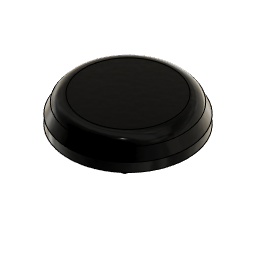
Suitcase v18 (Autodesk Fusion 360 archive; units mm, degrees)
design "LTE Antenna 202-4091"
Autodesk Fusion 360 part; units mm, degrees
(part 1 of 2)
sketch "Sketch1" plane through (0, 0, 0) normal (0, 1, 0) x (1, 0, 0)
  line L0 (0, 0) -> (0, -60.7821)
  line L1 (0, -15.2) -> (30, -15.2)
  line L2 (30, -15.2) -> (34.5, -5)
  line L3 (34.5, -5) -> (34.5, 0)
  line L4 (0, 0) -> (0, 30)
  line L5 (34.5, 0) -> (7.25, 0)
  line L6 (7.25, 0) -> (7.25, 19.3)
  line L7 (7.25, 19.3) -> (0, 19.3)
  dimension "d1" = 69
  dimension "d2" = 15.2
  dimension "d4" = 60
  dimension "d5" = 5
  dimension "d6" = 14.5
  dimension "d7" = 19.3
  constraint coincident L0.start L4.start
  constraint vertical L0
  constraint coincident L0 L1.start
  constraint perpendicular L0 L1
  constraint perpendicular L1 L3
  constraint parallel L0 L4
  constraint perpendicular L3 L5
  constraint perpendicular L5 L6
  constraint coincident L4 L7.end
  constraint perpendicular L4 L7
  constraint coincident L0.start L5
  measures "d2" distance of L0.start L1
  measures "d5" distance of L2.end L3.end
  measures "d7" distance of L5 L7
revolve "Revolve1" add sketch "Sketch1" angle 360 about axis through (0, 0, 0) along (0, 0, 1) makes body 1
fillet "Fillet1" radius 7 1 edges at (-27.9698, -10.8485, 15.2) on bodies 1
sketch "Sketch2" plane through (0, 0, -19.3) normal (0, 0, -1) x (1, 0, 0)
  circle A0 centre (0, 0) radius 7.25
  line L0 (2.75, 0) -> (2.75, 7.25)
  arc A1 (2.75, 7.25) -> (-2.75, 7.25) centre (0, 7.25) ccw
  line L1 (-2.75, 7.25) -> (-2.75, 0)
  arc A2 (-2.75, 0) -> (2.75, 0) centre (0, 0) ccw
  line L2 (0, 0) -> (0, 7.25) construction
  dimension "d11" = 5.5
  constraint tangent L0 A1
  constraint tangent A1 L1
  constraint parallel L0 L1
  constraint tangent L1 A2
  constraint tangent L0 A2
  constraint coincident A0 A1.centre
  constraint vertical L2
  constraint coincident A0.centre A2.centre
  measures "d11" distance of L0 L1
sketch "Sketch3" plane through (0, 0, 0) normal (0, 0, -1) x (1, 0, 0)
  circle A0 centre (0, 0) radius 7.25
  circle A1 centre (0, 0) radius 34.5
  line L0 (-7.25, 7.25) -> (7.25, 7.25)
  line L1 (7.25, 7.25) -> (7.25, -7.25)
  line L2 (7.25, -7.25) -> (-7.25, -7.25)
  line L3 (-7.25, -7.25) -> (-7.25, 7.25)
  circle A2 centre (0, 0) radius 7.25
  constraint horizontal L0
  constraint vertical L1
  constraint horizontal L2
  constraint vertical L3
  constraint tangent L1 A2
  constraint tangent L2 A2
  constraint tangent L3 A2
  constraint tangent L0 A2
extrude "Extrude1" add sketch "Sketch3" along normal blind 2.7 separate body contours A0 A2 | A0 L1 L2 A2 | A0 L0 L1 A2 | A0 L0 L3 A2 | A0 L2 L3 A2 makes body 2
extrude "Extrude2" cut sketch "Sketch2" against normal up to surface (19.3 mm away) contours A0 L0 L1 A2 | A0 L0 A1 L1 picked at (0, 2.4167) bodies 2 1
sketch "Sketch1 (2)" plane through (0, 0, 0) normal (0, 0, 1) x (1, 0, 0) in component "NUT"
  line L0 (11, -6.3509) -> (11, 6.3509)
  line L1 (11, 6.3509) -> (0, 12.7017)
  line L2 (0, 12.7017) -> (-11, 6.3509)
  line L3 (-11, 6.3509) -> (-11, -6.3509)
  line L4 (-11, -6.3509) -> (0, -12.7017)
  line L5 (0, -12.7017) -> (11, -6.3509)
  circle A0 centre (0, 0) radius 7.25
  dimension "d16" = 11
  dimension "d17" = 14.5
  constraint coincident A0.centre origin
  constraint vertical L0
  measures "d16" distance of A0.centre L5
  measures "d17" diameter of A0
extrude "Extrude1'" add sketch "Sketch1 (2)" against normal blind 5.6 separate body makes body 3 in component "NUT"
sketch "Sketch2 (2)" plane through (0, 0, 0) normal (0, 1, 0) x (1, 0, 0) in component "NUT"
  line L0 (0, 0) -> (10.6333, 0)
  line L1 (10.6333, 0) -> (13, 0)
  line L2 (13, 0) -> (13, -6.6)
  line L3 (13, -6.6) -> (12.2, -6.6)
  line L4 (12.2, -6.6) -> (12.2, -0.8)
  line L5 (12.2, -0.8) -> (7.5, -0.8)
  line L6 (7.5, -0.8) -> (7.5, 0)
  line L7 (0, 0) -> (0, -13)
  dimension "d20" = 6.6
  dimension "d21" = 15
  dimension "d22" = 26
  dimension "d23" = 0.8
  dimension "d24" = 0.8
  constraint coincident L0.start L7.start
  constraint horizontal L0
  constraint parallel L0 L1
  constraint perpendicular L1 L2
  constraint perpendicular L2 L3
  constraint perpendicular L3 L4
  constraint perpendicular L4 L5
  constraint coincident L0 L6.end
  constraint perpendicular L0 L6
  constraint perpendicular L0 L7
  measures "d20" distance of L1.end L2.end
  measures "d23" distance of L2 L4
  measures "d24" distance of L1 L5
revolve "Revolve1'" add sketch "Sketch2 (2)" angle 360 about axis through (0, 0, 0) along (0, 0, 1) bodies 3 in component "NUT"
sketch "Sketch3 (2)" plane through (0, 0, 0) normal (0, 1, 0) x (1, 0, 0) in component "NUT"
  line L0 (0, 0) -> (0, -11.559) construction
  line L1 (-9.7763, -5) -> (-1.7, -5)
  line L2 (-1.7, -5) -> (0, -6.7)
  line L3 (0, -6.7) -> (1.7, -5)
  line L4 (1.7, -5) -> (9.7763, -5)
  line L5 (9.7763, -5) -> (9.7763, -9.682)
  line L6 (9.7763, -9.682) -> (-9.7763, -9.682)
  line L7 (-9.7763, -9.682) -> (-9.7763, -5)
  dimension "d26" = 45
  dimension "d28" = 5
  dimension "d29" = 6.7
  dimension "d30" = 19.5526
  dimension "d31" = 4.682
  constraint coincident L0.start origin
  constraint vertical L0
  constraint horizontal L1
  constraint coincident L0 L2.end
  constraint perpendicular L0 L4
  constraint perpendicular L4 L5
  constraint perpendicular L5 L6
  constraint symmetric L0 L2 L3
  constraint collinear L1 L4
  constraint symmetric L0 L5 L7
  measures "d26" angle of L0 L2
  measures "d28" distance of L0.start L4
  measures "d29" distance of L0.start L2.end
  measures "d30" distance of L5 L7
  measures "d31" distance of L4 L6
extrude "Extrude2'" cut sketch "Sketch3 (2)" against normal blind 22 bodies 3 in component "NUT"
pattern_circular "C-Pattern1" count 4 over 360 about axis through (0, 0, 1.75) along (0, 0, 1) of "Extrude2'" in component "NUT"
component "NUT" placed x (1, 0, 0) y (0, 1, 0) z (0, 0, 1) at (0, 0, -10.4)
equation "d16 = 22 mm / 2"

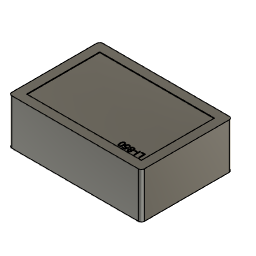
design "LICOR_850A"
Autodesk Fusion 360 part; units mm, degrees
sketch "Sketch1" plane through (0, 0, 0) normal (0, 0, 1) x (1, 0, 0)
  line L0 (0, 0) -> (222.3, 0)
  line L1 (222.3, 0) -> (222.3, 152.5)
  line L2 (222.3, 152.5) -> (0, 152.5)
  line L3 (0, 152.5) -> (0, 0)
  dimension "d1" = 222.3
  dimension "d2" = 152.5
  constraint horizontal L0
  constraint vertical L1
  constraint horizontal L2
  constraint vertical L3
  constraint coincident L0.start L3.end
  measures "d1" distance of L0.start L0.end
  measures "d2" distance of L0.start L2.end
extrude "Extrude1" add sketch "Sketch1" along normal blind 76.2
sketch "Sketch2" plane through (0, 0, 76.2) normal (0, 0, 1) x (-1, 0, 0)
  line L0 (0, -152.5) -> (0, 0)
  line L1 (0, 0) -> (-222.3, 0)
  line L2 (-222.3, 0) -> (-222.3, -152.5)
  line L3 (-222.3, -152.5) -> (0, -152.5)
fillet "Fillet1" radius 5 4 edges at (222.3, 0, 38.1) (0, 152.5, 38.1) (222.3, 152.5, 38.1) (0, 0, 38.1)
sketch "Sketch3" plane through (0, 0, 76.2) normal (0, 0, 1) x (-1, 0, 0)
  arc A0 (0, -5) -> (-5, 0) centre (-5, -5) ccw
  line L0 (-5, 0) -> (-217.3, 0)
  arc A1 (-217.3, 0) -> (-222.3, -5) centre (-217.3, -5) ccw
  line L1 (-222.3, -5) -> (-222.3, -147.5)
  arc A2 (-222.3, -147.5) -> (-217.3, -152.5) centre (-217.3, -147.5) ccw
  line L2 (-217.3, -152.5) -> (-5, -152.5)
  arc A3 (-5, -152.5) -> (0, -147.5) centre (-5, -147.5) ccw
  line L3 (0, -147.5) -> (0, -5)
  line L4 (-207.3, -15) -> (-207.3, -137.5)
  line L5 (-207.3, -137.5) -> (-15, -137.5)
  line L6 (-15, -137.5) -> (-15, -15)
  line L7 (-15, -15) -> (-207.3, -15)
  dimension "d7" = -15
extrude "Extrude2" cut sketch "Sketch3" against normal blind 1 contours L4 L5 L6 L7
sketch "Sketch4" plane through (0, 152.5, 0) normal (0, 1, 0) x (-1, 0, 0)
  line L0 (-217.3, 76.2) -> (-217.3, 0)
  line L1 (-217.3, 0) -> (-5, 0)
  line L2 (-5, 0) -> (-5, 76.2)
  line L3 (-5, 76.2) -> (-217.3, 76.2)
  line L4 (-135.3, 0) -> (-135.3, 76.2) construction
  circle A0 centre (-135.3, 30) radius 6
  line L5 (-111.15, 76.2) -> (-111.15, 0) construction
  circle A1 centre (-96, 30) radius 6
  line L6 (-201.4, 35) -> (-182.4, 35)
  line L7 (-182.4, 35) -> (-182.4, 25.3) construction
  line L8 (-182.4, 25.3) -> (-201.4, 25.3)
  line L9 (-201.4, 25.3) -> (-201.4, 35) construction
  line L10 (-201.4, 35) -> (-199.4, 25.3)
  line L11 (-182.4, 35) -> (-184.4, 25.3)
  circle A2 centre (-176.9, 30.15) radius 2.5
  line L12 (-191.9, 35) -> (-191.9, 25.3) construction
  line L13 (-191.9, 30.15) -> (-176.9, 30.15) construction
  circle A3 centre (-206.9, 30.15) radius 2.5
  line L14 (-81, 16.3) -> (-25.17, 16.3)
  line L15 (-25.17, 16.3) -> (-25.17, 9.5)
  line L16 (-25.17, 9.5) -> (-81, 9.5)
  line L17 (-81, 9.5) -> (-81, 16.3)
  line L18 (0, 0) -> (0, 76.2)
  point P0 (-222.3, 76.2)
  dimension "d10" = 87
  dimension "d11" = 30
  dimension "d12" = 12
  dimension "d13" = 19
  dimension "d14" = 9.7
  dimension "d15" = 2
  dimension "d16" = 2
  dimension "d17" = 5
  dimension "d18" = 15
  dimension "d19" = 35
  dimension "d20" = 45.4
  dimension "d21" = 55.83
  dimension "d22" = 6.8
  dimension "d23" = 16.3
  dimension "d24" = 81
  dimension "d25" = 96
  dimension "d26" = 30
  dimension "d27" = 12
  constraint coincident L1 L4.start
  constraint coincident L3 L4.end
  constraint perpendicular L3 L4
  constraint midpoint L3 L5.start
  constraint midpoint L1 L5.end
  constraint horizontal L6
  constraint vertical L7
  constraint horizontal L8
  constraint vertical L9
  constraint coincident L8 L10.end
  constraint coincident L8 L11.end
  constraint midpoint L6 L12.start
  constraint midpoint L8 L12.end
  constraint midpoint L12 L13.start
  constraint coincident A2.centre L13.end
  constraint horizontal L13
  constraint symmetric A2 L12 A3
  constraint coincident L4 A0.centre
  constraint horizontal L14
  constraint vertical L15
  constraint horizontal L16
  constraint vertical L17
  measures "d10" distance of L4 P0
  measures "d11" distance of L1 A0.centre
  measures "d12" diameter of A0
  measures "d13" distance of L7 L9
  measures "d14" distance of L6 L8
  measures "d15" distance of L7.end L11.end
  measures "d16" distance of L8.end L10.end
  measures "d17" diameter of A2
  measures "d18" distance of A2.centre L12
  measures "d19" distance of L4.start L6
  measures "d20" horizontal distance of P0 A2.centre
  measures "d21" distance of L15 L17
  measures "d22" distance of L14.start L16.end
  measures "d23" distance of L1 L14
  measures "d24" distance of L18.start L17
  measures "d25" distance of A1.centre L18
  measures "d26" distance of L1 A1.centre
  measures "d27" diameter of A1
extrude "Extrude3" cut sketch "Sketch4" against normal blind 10 contours L14 L15 L16 L17
extrude "Extrude4" add sketch "Sketch4" along normal blind 25 contours A0 | A1
extrude "Extrude5" add sketch "Sketch4" along normal blind 2.66 contours L6 L8 L10 L11 | A2 | A3
sketch "Sketch5" plane through (0, 0, 76.2) normal (0, 0, 1) x (-1, 0, 0)
  line L0 (-201.1791, -42.0416) -> (-144.1791, -42.0416) construction
  line L1 (-144.1791, -42.0416) -> (-144.1791, -18.0416) construction
  line L2 (-144.1791, -18.0416) -> (-201.1791, -18.0416) construction
  line L3 (-201.1791, -18.0416) -> (-201.1791, -42.0416) construction
  dimension "d34" = 10
  text T0 "LI-850" font "Arial" height 10 align left top in box 57 x 24 at (-201.1791, -42.0416) x (1, 0) y (0, 1) spacing 1 kerned
extrude "Extrude6" cut sketch "Sketch5" against normal blind 2 text T0
equation "d26 = d11"
equation "d27 = d12"

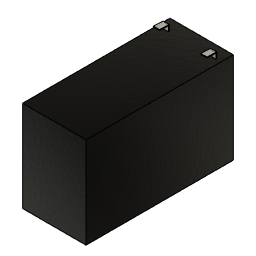
design "RS PRO 12V Sealed Lead Acid Battery - 9Ah"
Autodesk Fusion 360 part; units mm, degrees
sketch "Sketch1" plane through (0, 0, 0) normal (0, 0, 1) x (1, 0, 0)
  line L0 (32.5, 75.5) -> (-32.5, 75.5)
  line L1 (-32.5, 75.5) -> (-32.5, -75.5)
  line L2 (-32.5, -75.5) -> (32.5, -75.5)
  line L3 (32.5, -75.5) -> (32.5, 75.5)
  line L4 (32.5, 75.5) -> (-32.5, -75.5) construction
  line L5 (-32.5, 75.5) -> (32.5, -75.5) construction
  dimension "d1" = 65
  dimension "d2" = 151
  constraint horizontal L0
  constraint perpendicular L0 L1
  constraint parallel L0 L2
  constraint parallel L1 L3
  constraint coincident L4 origin
  constraint coincident L5 origin
  measures "d1" distance of L1.end L2.end
  measures "d2" distance of L0.end L1.end
extrude "Extrude1" add sketch "Sketch1" along normal blind 93.5 makes body 1
ref_plane "WorkPlane1" through (27.5, 0, 46.75) normal (1, 0, 0) x (0, 1, 0)
sketch "Sketch2" plane through (27.5, 0, 46.75) normal (1, 0, 0) x (0, 1, 0)
  line L0 (63.5, 46.75) -> (63.5, 52.75)
  line L1 (63.5, 52.75) -> (53.5, 53.25)
  line L2 (-75.5, -46.75) -> (75.5, -46.75)
  line L3 (-75.5, 46.75) -> (75.5, 46.75)
  line L4 (53.5, 53.25) -> (53.46, 52.451)
  line L5 (53.46, 52.451) -> (62.7, 51.989)
  line L6 (62.7, 51.989) -> (62.7, 46.75)
  dimension "d6" = 100
  dimension "d7" = 10
  dimension "d8" = 12
  dimension "d9" = 6
  dimension "d10" = 0.8
  dimension "d11" = 0.8
  constraint vertical L0
  constraint coincident L0.start L3
  constraint perpendicular L1 L4
  constraint perpendicular L4 L5
  constraint coincident L3 L6.end
  constraint perpendicular L3 L6
  measures "d6" distance of L1.end L2
  measures "d7" distance of L0 L1.end
  measures "d8" distance of L0 L3.end
  measures "d9" distance of L0.start L0.end
  measures "d10" distance of L0 L6
  measures "d11" distance of L1 L5
extrude "Extrude2" add sketch "Sketch2" against normal blind 6.35 separate body makes body 2
mirror "Mirror1" about plane through (0, 0, 0) normal (1, 0, 0) of "Extrude2" makes body 3

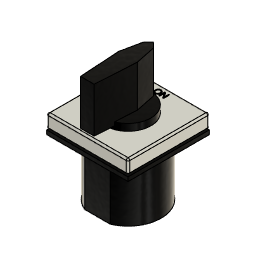
design "RS-PRO_SWITCH"
Autodesk Fusion 360 part; units mm, degrees
sketch "Sketch1" plane through (0, 0, 0) normal (0, 0, 1) x (1, 0, 0)
  line L0 (24, 24) -> (-24, 24)
  line L1 (-24, 24) -> (-24, -24)
  line L2 (-24, -24) -> (24, -24)
  line L3 (24, -24) -> (24, 24)
  line L4 (24, 24) -> (-24, -24) construction
  line L5 (-24, 24) -> (24, -24) construction
  circle A0 centre (0, 0) radius 6
  circle A1 centre (-18, 18) radius 2.5
  circle A2 centre (18, 18) radius 2.5
  circle A3 centre (18, -18) radius 2.5
  circle A4 centre (-18, -18) radius 2.5
  line L6 (-18, 18) -> (18, 18)
  line L7 (18, 18) -> (18, -18)
  line L8 (18, -18) -> (-18, -18)
  line L9 (-18, -18) -> (-18, 18)
  circle A5 centre (0, 0) radius 19.5
  circle A6 centre (0, 0) radius 13.5
  dimension "d1" = 48
  dimension "d2" = 48
  dimension "d3" = 12
  dimension "d4" = 5
  dimension "d5" = 5
  dimension "d6" = 5
  dimension "d7" = 5
  dimension "d8" = 36
  dimension "d9" = 39
  dimension "d10" = 27
  constraint horizontal L0
  constraint perpendicular L0 L1
  constraint parallel L0 L2
  constraint parallel L1 L3
  constraint coincident L4 A0.centre
  constraint coincident L5 A0.centre
  constraint coincident A0.centre A5.centre
  constraint horizontal L6
  constraint vertical L7
  constraint horizontal L8
  constraint vertical L9
  constraint coincident L5 A3.centre
  constraint coincident L5 A1.centre
  constraint coincident L4 A4.centre
  constraint coincident A1.centre L6.start
  constraint coincident A2.centre L7
  constraint coincident A2.centre L6.end
  constraint coincident A3.centre L7.end
  constraint coincident A4.centre L8.end
  constraint concentric A0 A5
  measures "d1" distance of L1.end L2.end
  measures "d2" distance of L0.end L1.end
  measures "d3" diameter of A0
  measures "d4" diameter of A1
  measures "d5" diameter of A2
  measures "d6" diameter of A4
  measures "d7" diameter of A3
  measures "d8" distance of A4.centre L7
  measures "d9" diameter of A5
  measures "d10" diameter of A6
extrude "Extrude1" add sketch "Sketch1" against normal blind 33 contours A0 | L6 L7 L8 L9 A5 | L9 A5 | L7 A5 | A6 makes body 1
extrude "Extrude2" add sketch "Sketch1" along normal blind 2.4 contours L0 L1 L2 L3 | A0 | A1 L6 L9 A5 | L6 A5 | L6 L7 L8 L9 A5 | L9 A5 | A2 L6 L7 A5 | A4 L8 L9 A5 | L7 A5 | L8 A5 | A3 L7 L8 A5 | A6 bodies 1
sketch "Sketch2" plane through (0, 0, 2.4) normal (0, 0, 1) x (-1, 0, 0)
  circle A0 centre (18, -18) radius 2.5
  circle A1 centre (-18, 18) radius 2.5
  circle A2 centre (18, 18) radius 2.5
  circle A3 centre (-18, -18) radius 2.5
  line L0 (-24, 24) -> (-24, -24)
  line L1 (-24, -24) -> (24, -24)
  line L2 (24, -24) -> (24, 24)
  line L3 (24, 24) -> (-24, 24)
  line L4 (-24, -24) -> (24, 24)
  circle A4 centre (0, 0) radius 6
  circle A5 centre (-18, -18) radius 2.5
  circle A6 centre (18, -18) radius 2.5
  circle A7 centre (-18, 18) radius 2.5
  circle A8 centre (18, 18) radius 2.5
extrude "Extrude3" add sketch "Sketch2" along normal blind 1.5 contours A0 A6 | A1 A7 | A2 L4 A8 | A2 L4 A8 | L4 A4 | L4 A4 | A3 L4 A5 | A3 L4 A5 bodies 1
sketch "Sketch3" plane through (0, 0, 3.9) normal (0, 0, 1) x (-1, 0, 0)
  circle A0 centre (18, 18) radius 2.5
  line L0 (24, -24) -> (24, 24)
  line L1 (24, 24) -> (-24, 24)
  line L2 (-24, 24) -> (-24, -24)
  line L3 (-24, -24) -> (24, -24)
extrude "Extrude4" add sketch "Sketch3" along normal blind 7.3 separate body contours A0 | L0 L1 L2 L3 makes body 2
sketch "Sketch4" plane through (0, 0, 11.2) normal (0, 0, 1) x (-1, 0, 0)
  line L0 (-24, -24) -> (24, -24)
  line L1 (24, -24) -> (24, 24)
  line L2 (24, 24) -> (-24, 24)
  line L3 (-24, 24) -> (-24, -24)
  line L4 (5.5, -15) -> (-5.5, -15)
  line L5 (-5.5, -15) -> (-5.5, 24)
  line L6 (-5.5, 24) -> (5.5, 24)
  line L7 (5.5, 24) -> (5.5, -15)
  line L8 (0, 0) -> (0, -18) construction
  line L9 (24, 24) -> (-24, 24)
  line L10 (0, 0) -> (-5.5, 0) construction
  line L11 (0, -15) -> (-5.5, -9.5)
  line L12 (-5.5, 0) -> (-3, -12)
  line L13 (-5.5, 0) -> (-4, 24)
  line L14 (5.5, 0) -> (4, 24)
  line L15 (5.5, 0) -> (3, -12)
  line L16 (0, -15) -> (5.5, -9.5)
  dimension "d19" = 39
  dimension "d20" = 11
  dimension "d21" = 1.5
  dimension "d22" = 45
  dimension "d23" = 3
  constraint horizontal L4
  constraint vertical L5
  constraint horizontal L6
  constraint vertical L7
  constraint coincident L8.start L10.start
  constraint parallel L7 L8
  constraint symmetric L5 L7 L8
  constraint collinear L6 L9
  constraint coincident L5 L10.end
  constraint perpendicular L5 L10
  constraint midpoint L4 L11.start
  constraint coincident L5 L11.end
  constraint coincident L11 L12.end
  constraint coincident L9 L13.end
  constraint coincident L6 L13.end
  constraint symmetric L8 L10.end L14.start
  constraint symmetric L8 L11.start L16.start
  constraint symmetric L8 L11.end L16.end
  constraint symmetric L8 L12.end L15.end
  constraint symmetric L8 L13.end L14.end
  measures "d19" distance of L4 L6
  measures "d20" distance of L5 L7
  measures "d21" distance of L5.end L13.end
  measures "d22" angle of L4 L11
  measures "d23" distance of L4 L12.end
sketch "Sketch6" plane through (0, 0, 11.2) normal (0, 0, 1) x (-1, 0, 0)
  line L0 (-24, 24) -> (-24, -24)
  line L1 (-24, -24) -> (24, -24)
  line L2 (24, -24) -> (24, 24)
  line L3 (24, 24) -> (-24, 24)
  circle A0 centre (0, 0) radius 13.5
extrude "Extrude6" add sketch "Sketch6" along normal blind 4 separate body contours A0 makes body 3
extrude "Extrude7" add sketch "Sketch4" along normal blind 26.5 from surface at 2 contours L2 L6 L9 L11 L12 L13 L14 L15 L16 bodies 3
sketch "Sketch7" plane through (0, 0, 11.2) normal (0, 0, 1) x (-1, 0, 0)
  line L0 (-24, -24) -> (24, -24)
  line L1 (24, -24) -> (24, 24)
  line L2 (24, 24) -> (-24, 24)
  line L3 (-24, 24) -> (-24, -24)
  line L4 (3.6415, -14.8993) -> (-9.9533, -14.8993) construction
  line L5 (-9.9533, -14.8993) -> (-9.9533, -21.3648) construction
  line L6 (-9.9533, -21.3648) -> (3.6415, -21.3648) construction
  line L7 (3.6415, -21.3648) -> (3.6415, -14.8993) construction
  line L8 (22.4194, 12.149) -> (9.4194, 12.149) construction
  line L9 (9.4194, 12.149) -> (9.4194, -0.851) construction
  line L10 (9.4194, -0.851) -> (22.4194, -0.851) construction
  line L11 (22.4194, -0.851) -> (22.4194, 12.149) construction
  dimension "d31" = 3.5
  dimension "d32" = 3.5
  text T0 "ON\n" font "Arial" height 3.5 align left top in box 13.5948 x 6.4654 at (3.6415, -14.8993) x (-1, 0) y (0, -1) spacing 1 kerned
  text T1 "OFF" font "Arial" height 3.5 align left top in box 13 x 13 at (22.4194, 12.149) x (-1, 0) y (0, -1) spacing 1 kerned
extrude "Extrude8" cut sketch "Sketch7" against normal blind 0.2 text T0 T1 bodies 3 2
fillet "Fillet1" radius 1 8 edges at (-24, 0, 11.2) (0, 24, 11.2) (24, 0, 11.2) (0, -24, 11.2) (-24, -24, 7.55) (-24, 24, 7.55) (24, 24, 7.55) (24, -24, 7.55) on bodies 2

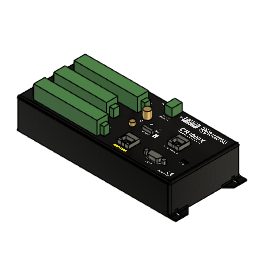
design "CR1000X"
Autodesk Fusion 360 part; units mm, degrees
sketch "Sketch1" plane through (0, 0, 0) normal (0, 0, 1) x (1, 0, 0)
  line L0 (110, 51) -> (-110, 51)
  line L1 (-110, 51) -> (-110, -51)
  line L2 (-110, -51) -> (110, -51)
  line L3 (110, -51) -> (110, 51)
  line L4 (110, 51) -> (-110, -51) construction
  line L5 (-110, 51) -> (110, -51) construction
  line L6 (110, 51) -> (119, 51)
  line L7 (119, 51) -> (119, 24)
  line L8 (119, 24) -> (110, 24)
  line L9 (110, 24) -> (110, 51)
  line L10 (110, 24) -> (119, 33)
  line L11 (110, 38.9) -> (114.75, 38.9)
  arc A0 (114.75, 38.9) -> (114.75, 42.8) centre (114.75, 40.85) ccw
  line L12 (114.75, 42.8) -> (110, 42.8)
  arc A1 (110, 42.8) -> (110, 38.9) centre (110, 40.85) ccw
  line L13 (110, 40.85) -> (114.75, 40.85) construction
  line L14 (0, 0) -> (110, 0) construction
  line L15 (0, 0) -> (0, 51) construction
  line L16 (110, -24) -> (110, -51)
  line L17 (110, -40.85) -> (114.75, -40.85) construction
  arc A2 (114.75, -42.8) -> (114.75, -38.9) centre (114.75, -40.85) ccw
  line L18 (119, -24) -> (110, -24)
  line L19 (119, -51) -> (119, -24)
  arc A3 (110, -38.9) -> (110, -42.8) centre (110, -40.85) ccw
  line L20 (110, -51) -> (119, -51)
  line L21 (110, -24) -> (119, -33)
  line L22 (110, -38.9) -> (114.75, -38.9)
  line L23 (114.75, -42.8) -> (110, -42.8)
  line L24 (-110, 29) -> (-119.6, 29)
  line L25 (-119.6, 29) -> (-119.6, -29)
  line L26 (-119.6, -29) -> (-110, -29)
  line L27 (-110, -29) -> (-110, 29)
  line L28 (-110, 29) -> (-119.6, 21)
  line L29 (-110, -29) -> (-119.6, -21)
  line L30 (-119.6, 11.1) -> (-115.13, 11.1)
  arc A4 (-115.13, 11.1) -> (-115.13, 15) centre (-115.13, 13.05) ccw
  line L31 (-115.13, 15) -> (-119.6, 15)
  arc A5 (-119.6, 15) -> (-119.6, 11.1) centre (-119.6, 13.05) ccw
  line L32 (-119.6, 13.05) -> (-115.13, 13.05) construction
  arc A6 (-119.6, -11.1) -> (-119.6, -15) centre (-119.6, -13.05) ccw
  line L33 (-119.6, -13.05) -> (-115.13, -13.05) construction
  arc A7 (-115.13, -15) -> (-115.13, -11.1) centre (-115.13, -13.05) ccw
  line L34 (-119.6, -11.1) -> (-115.13, -11.1)
  line L35 (-115.13, -15) -> (-119.6, -15)
  dimension "d1" = 220
  dimension "d2" = 102
  dimension "d5" = 9
  dimension "d6" = 27
  dimension "d7" = 18
  dimension "d8" = 8.2
  dimension "d9" = 3.9
  dimension "d10" = 4.75
  dimension "d11" = 9.6
  dimension "d12" = 58
  dimension "d13" = 8
  dimension "d14" = 3.9
  dimension "d15" = 14
  dimension "d16" = 4.47
  constraint horizontal L0
  constraint perpendicular L0 L1
  constraint parallel L0 L2
  constraint parallel L1 L3
  constraint coincident L4 L14.start
  constraint coincident L5 L14.start
  constraint coincident L14.start L15.start
  constraint horizontal L6
  constraint vertical L7
  constraint horizontal L8
  constraint vertical L9
  constraint coincident L7 L10.end
  constraint tangent L11 A0
  constraint tangent A0 L12
  constraint parallel L11 L12
  constraint tangent L12 A1
  constraint tangent L11 A1
  constraint perpendicular L9 L13
  constraint coincident L3 A1.centre
  constraint midpoint L3 L14.end
  constraint midpoint L0 L15.end
  constraint symmetric L0.start L14 L2.end
  constraint symmetric L6.end L14 L19.start
  constraint symmetric L7.end L14 L18.start
  constraint symmetric L8.end L14 L16.start
  constraint symmetric L10.end L14 L21.end
  constraint symmetric L11.start L14 A3.start
  constraint symmetric L11.end L14 A2.end
  constraint symmetric A0.end L14 A2.start
  constraint symmetric L12.end L14 A3.end
  constraint symmetric A0 L14 A2
  constraint symmetric A1 L14 A3
  constraint horizontal L24
  constraint vertical L25
  constraint horizontal L26
  constraint vertical L27
  constraint coincident L1 L24.start
  constraint symmetric L14 L24 L26
  constraint coincident L25 L28.end
  constraint coincident L25 L29.end
  constraint symmetric L14 L28 L29
  constraint tangent L30 A4
  constraint tangent A4 L31
  constraint parallel L30 L31
  constraint tangent L31 A5
  constraint tangent L30 A5
  constraint perpendicular L25 L32
  constraint coincident L25 A5.centre
  constraint symmetric L14 L30.start A6.start
  constraint symmetric L14 L30.end A7.end
  constraint symmetric L14 A4.end A7.start
  constraint symmetric L14 L31.end A6.end
  constraint symmetric L14 A4 A7
  constraint symmetric L14 A5 A6
  measures "d1" distance of L1.end L2.end
  measures "d2" distance of L0 L2
  measures "d5" distance of L0.start L6.end
  measures "d6" distance of L6.end L7.end
  measures "d7" distance of L6.end L10.end
  measures "d8" distance of L6 L12
  measures "d9" distance of L11 L12
  measures "d10" distance of L3 A0.centre
  measures "d11" distance of L25 L27
  measures "d12" distance of L24 L26
  measures "d13" distance of L24.end L28.end
  measures "d14" distance of L30 L31
  measures "d15" distance of L24.start L31
  measures "d16" distance of L25 A4.centre
extrude "Extrude1" add sketch "Sketch1" along normal blind 43 contours L0 L1 L2 L3 L9 A1 L16 A3 L27 | L3 L9 A1 | L3 L16 A3 makes body 1
sketch "Sketch2" plane through (110, 0, 0) normal (1, 0, 0) x (0, 1, 0)
  line L0 (-51, 0) -> (51, 0)
  line L1 (51, 0) -> (51, 43)
  line L2 (51, 43) -> (-51, 43)
  line L3 (-51, 43) -> (-51, 0)
extrude "Extrude2" add sketch "Sketch1" along normal blind 1.6 contours L3 L6 L7 L9 L10 L11 A0 L12 | L1 L25 L27 L28 L29 L30 A4 L31 A7 L34 L35 | L3 L16 A2 L19 L20 L21 L22 L23 bodies 1
extrude "Extrude3" cut sketch "Sketch1" along normal blind 6 contours L3 L9 A1 | L3 L16 A3 bodies 1
fillet "Fillet2" radius 2.8 8 edges at (110, 51, 22.3) (110, -51, 22.3) (-110, -51, 21.5) (-110, 0, 43) (-110, 51, 21.5) (0, 51, 43) (0, -51, 43) (110, 0, 43) on bodies 1
fillet "Fillet1" radius 1.6 5 edges at (110, -46.9, 1.6) (110, -31.45, 1.6) (110, 31.45, 1.6) (110, 46.9, 1.6) (-110, 0, 1.6) on bodies 1
sketch "Sketch3" plane through (0, 0, 43) normal (0, 0, 1) x (-1, 0, 0)
  line L0 (107.2, -48.2) -> (107.2, 48.2)
  line L1 (107.2, 48.2) -> (-107.2, 48.2)
  line L2 (-107.2, 48.2) -> (-107.2, -48.2)
  line L3 (-107.2, -48.2) -> (107.2, -48.2)
  line L4 (-110, -51) -> (110, -51)
  line L5 (110, -51) -> (110, 51)
  line L6 (-110, 51) -> (-110, -51)
  line L7 (110, 51) -> (-110, 51)
  line L8 (-19.39, -41) -> (-31.5, -41)
  line L9 (-31.5, -41) -> (-31.5, -32.3)
  line L10 (-31.5, -32.3) -> (-19.39, -32.3)
  line L11 (-19.39, -32.3) -> (-19.39, -41)
  line L12 (-23.2635, -0.0276) -> (-36.8497, -0.0276)
  line L13 (-36.8497, -0.0276) -> (-36.8497, 3.4029)
  line L14 (-36.8497, 3.4029) -> (-23.2635, 3.4029)
  line L15 (-23.2635, 3.4029) -> (-23.2635, -0.0276)
  line L16 (-61, -12.3) -> (-77, -12.3)
  line L17 (-77, -12.3) -> (-77, 4.7)
  line L18 (-77, 4.7) -> (-61, 4.7)
  line L19 (-61, 4.7) -> (-61, -12.3)
  line L20 (-90.2257, 11.596) -> (-97.7934, 11.596)
  line L21 (-97.7934, 11.596) -> (-97.7934, 14.801)
  line L22 (-97.7934, 14.801) -> (-90.2257, 14.801)
  line L23 (-90.2257, 14.801) -> (-90.2257, 11.596)
  line L24 (-22.5, 21.2) -> (-38.5, 21.2)
  line L25 (-38.5, 21.2) -> (-38.5, 38.2)
  line L26 (-38.5, 38.2) -> (-22.5, 38.2)
  line L27 (-22.5, 38.2) -> (-22.5, 21.2)
  line L28 (91.5, -29.8) -> (0.5, -29.8)
  line L29 (0.5, -29.8) -> (0.5, -13.8)
  line L30 (0.5, -13.8) -> (91.5, -13.8)
  line L31 (91.5, -13.8) -> (91.5, -29.8)
  line L32 (91.5, -0.8) -> (15.9, -0.8)
  line L33 (15.9, -0.8) -> (15.9, 15.2)
  line L34 (15.9, 15.2) -> (91.5, 15.2)
  line L35 (91.5, 15.2) -> (91.5, -0.8)
  line L36 (91.5, 28.2) -> (0.5, 28.2)
  line L37 (0.5, 28.2) -> (0.5, 44.2)
  line L38 (0.5, 44.2) -> (91.5, 44.2)
  line L39 (91.5, 44.2) -> (91.5, 28.2)
  circle A0 centre (-12.5, -15) radius 4.75
  circle A1 centre (-10.5284, 4.5374) radius 3.5
  line L40 (97, -27) -> (-5, -27)
  line L41 (-5, -27) -> (-5, -19)
  line L42 (-5, -19) -> (97, -19)
  line L43 (97, -19) -> (97, -27)
  line L44 (96.7037, 2.3694) -> (10.018, 2.3694)
  line L45 (10.018, 2.3694) -> (10.018, 10.9549)
  line L46 (10.018, 10.9549) -> (96.7037, 10.9549)
  line L47 (96.7037, 10.9549) -> (96.7037, 2.3694)
  line L48 (96.7037, 31.5878) -> (-4.9374, 31.5878)
  line L49 (-4.9374, 31.5878) -> (-4.9374, 39.7578)
  line L50 (-4.9374, 39.7578) -> (96.7037, 39.7578)
  line L51 (96.7037, 39.7578) -> (96.7037, 31.5878)
  line L52 (-60.4037, 28.8936) -> (-61.6094, 33.5058)
  line L53 (-63.5444, 35) -> (-74.4822, 35)
  line L54 (-76.4084, 33.5381) -> (-77.7111, 28.875)
  line L55 (-75.7773, 26.3369) -> (-62.3311, 26.3877)
  arc A2 (-62.3311, 26.3877) -> (-60.4037, 28.8936) centre (-62.3387, 28.3877) ccw
  arc A3 (-77.7111, 28.875) -> (-75.7773, 26.3369) centre (-75.7849, 28.3369) ccw
  arc A4 (-74.4822, 35) -> (-76.4084, 33.5381) centre (-74.4822, 33) ccw
  arc A5 (-61.6094, 33.5058) -> (-63.5444, 35) centre (-63.5444, 33) ccw
  line L56 (-58.2072, 28.1876) -> (-55.4144, 28.1751)
  line L57 (-55.4144, 28.1751) -> (-54.0072, 30.5876)
  line L58 (-54.0072, 30.5876) -> (-55.3928, 33.0124)
  line L59 (-55.3928, 33.0124) -> (-58.1856, 33.0249)
  line L60 (-58.1856, 33.0249) -> (-59.5928, 30.6124)
  line L61 (-59.5928, 30.6124) -> (-58.2072, 28.1876)
  line L62 (-83.3239, 28.1243) -> (-80.4215, 28.0485)
  line L63 (-80.4215, 28.0485) -> (-78.9047, 30.5243)
  line L64 (-78.9047, 30.5243) -> (-80.2903, 33.0757)
  line L65 (-80.2903, 33.0757) -> (-83.1928, 33.1515)
  line L66 (-83.1928, 33.1515) -> (-84.7096, 30.6757)
  line L67 (-84.7096, 30.6757) -> (-83.3239, 28.1243)
  line L68 (-63, -7) -> (-75.7219, -7)
  line L69 (-75.7219, -7) -> (-75.7219, 1.2588)
  line L70 (-75.7219, 1.2588) -> (-63, 1.2588)
  line L71 (-63, 1.2588) -> (-63, -7)
  line L72 (-66.1152, 1.2588) -> (-72.5, 1.2588)
  line L73 (-72.5, 1.2588) -> (-72.5, 3)
  line L74 (-72.5, 3) -> (-66.1152, 3)
  line L75 (-66.1152, 3) -> (-66.1152, 1.2588)
  line L76 (-67.5, 3) -> (-71.2537, 3)
  line L77 (-71.2537, 3) -> (-71.2537, 4.0794)
  line L78 (-71.2537, 4.0794) -> (-67.5, 4.0794)
  line L79 (-67.5, 4.0794) -> (-67.5, 3)
  line L80 (-24, 27) -> (-37, 27)
  line L81 (-37, 27) -> (-37, 35)
  line L82 (-37, 35) -> (-24, 35)
  line L83 (-24, 35) -> (-24, 27)
  line L84 (-27, 35) -> (-33.579, 35)
  line L85 (-33.579, 35) -> (-33.579, 36.7205)
  line L86 (-33.579, 36.7205) -> (-27, 36.7205)
  line L87 (-27, 36.7205) -> (-27, 35)
  line L88 (-28.1815, 36.7205) -> (-32.7185, 36.7205)
  line L89 (-32.7185, 36.7205) -> (-32.7185, 38.0112)
  line L90 (-32.7185, 38.0112) -> (-28.1815, 38.0112)
  line L91 (-28.1815, 38.0112) -> (-28.1815, 36.7205)
  line L92 (-75.7792, 26.8369) -> (-62.333, 26.8877)
  arc A6 (-62.333, 26.8877) -> (-60.8874, 28.7671) centre (-62.3387, 28.3877) ccw
  line L93 (-60.8874, 28.7671) -> (-62.0931, 33.3794)
  arc A7 (-62.0931, 33.3794) -> (-63.5444, 34.5) centre (-63.5444, 33) ccw
  line L94 (-63.5444, 34.5) -> (-74.4822, 34.5)
  arc A8 (-74.4822, 34.5) -> (-75.9268, 33.4036) centre (-74.4822, 33) ccw
  line L95 (-75.9268, 33.4036) -> (-77.2296, 28.7405)
  arc A9 (-77.2296, 28.7405) -> (-75.7792, 26.8369) centre (-75.7849, 28.3369) ccw
  line L96 (-20, -47) -> (-30.5289, -47)
  line L97 (-30.5289, -47) -> (-30.5289, -32.3)
  line L98 (-30.5289, -32.3) -> (-20, -32.3)
  line L99 (-20, -32.3) -> (-20, -47)
  point P0 (-56.8, 30.6)
  point P1 (-81.8071, 30.6)
  dimension "d25" = 91
  dimension "d26" = 16
  dimension "d27" = 75.6
  dimension "d28" = 16
  dimension "d29" = 91
  dimension "d30" = 18.5
  dimension "d31" = 21.2
  dimension "d32" = 29
  dimension "d33" = 29
  dimension "d34" = 16
  dimension "d35" = 9.5
  dimension "d36" = 7
  dimension "d37" = 12.11
  dimension "d38" = 8.7
  dimension "d39" = 10
  dimension "d40" = 78.5
  dimension "d41" = 17
  dimension "d42" = 16
  dimension "d43" = 38.7
  dimension "d44" = 33
  dimension "d45" = 17
  dimension "d46" = 16
  dimension "d47" = 71.5
  dimension "d48" = 12.8
  dimension "d50" = 2
  dimension "d51" = 2
  dimension "d56" = -0.5
  constraint horizontal L8
  constraint vertical L9
  constraint horizontal L10
  constraint vertical L11
  constraint horizontal L12
  constraint vertical L13
  constraint horizontal L14
  constraint vertical L15
  constraint horizontal L16
  constraint vertical L17
  constraint horizontal L18
  constraint vertical L19
  constraint horizontal L20
  constraint vertical L21
  constraint horizontal L22
  constraint vertical L23
  constraint horizontal L24
  constraint vertical L25
  constraint horizontal L26
  constraint vertical L27
  constraint horizontal L28
  constraint vertical L29
  constraint horizontal L30
  constraint vertical L31
  constraint horizontal L32
  constraint vertical L33
  constraint horizontal L34
  constraint vertical L35
  constraint horizontal L36
  constraint vertical L37
  constraint horizontal L38
  constraint vertical L39
  constraint collinear L31 L35
  constraint collinear L35 L39
  constraint horizontal L40
  constraint vertical L41
  constraint horizontal L42
  constraint vertical L43
  constraint horizontal L44
  constraint vertical L45
  constraint horizontal L46
  constraint vertical L47
  constraint horizontal L48
  constraint vertical L49
  constraint horizontal L50
  constraint vertical L51
  constraint horizontal L53
  constraint tangent L52 A2
  constraint tangent L55 A2
  constraint tangent L55 A3
  constraint tangent L54 A3
  constraint tangent L54 A4
  constraint tangent L53 A4
  constraint equal A3 A4
  constraint tangent L52 A5
  constraint tangent L53 A5
  constraint equal A3 A5
  constraint horizontal L68
  constraint vertical L69
  constraint horizontal L70
  constraint vertical L71
  constraint horizontal L72
  constraint vertical L73
  constraint horizontal L74
  constraint vertical L75
  constraint coincident L70 L72.start
  constraint horizontal L76
  constraint vertical L77
  constraint horizontal L78
  constraint vertical L79
  constraint coincident L74 L76.start
  constraint horizontal L80
  constraint vertical L81
  constraint horizontal L82
  constraint vertical L83
  constraint horizontal L84
  constraint vertical L85
  constraint horizontal L86
  constraint vertical L87
  constraint coincident L82 L84.start
  constraint horizontal L88
  constraint vertical L89
  constraint horizontal L90
  constraint vertical L91
  constraint coincident L86 L88.start
  constraint horizontal L96
  constraint vertical L97
  constraint horizontal L98
  constraint vertical L99
  constraint coincident L10 L97.end
  measures "d25" distance of L29 L31
  measures "d26" distance of L28 L30
  measures "d27" distance of L32.start L32.end
  measures "d28" distance of L32.start L34.end
  measures "d29" distance of L36.start L36.end
  measures "d30" distance of L5 L31
  measures "d31" distance of L4 L28
  measures "d32" distance of L28 L32
  measures "d33" distance of L32 L36
  measures "d34" distance of L36 L38
  measures "d35" diameter of A0
  measures "d36" diameter of A1
  measures "d37" distance of L8.start L8.end
  measures "d38" distance of L8.end L9.end
  measures "d39" distance of L4 L8
  measures "d40" distance of L6 L9
  measures "d41" distance of L16.end L17.end
  measures "d42" distance of L16.start L16.end
  measures "d43" distance of L4 L16
  measures "d44" distance of L6 L17
  measures "d45" distance of L24.end L25.end
  measures "d46" distance of L24.start L24.end
  measures "d47" distance of L6 L25
  measures "d48" distance of L7 L26
  measures "d50" radius of A2
  measures "d51" radius of A3
extrude "Extrude4" add sketch "Sketch3" along normal blind 19.7 separate body contours L28 L29 L31 L40 | L29 L31 L40 L42 | L29 L30 L31 L42 | L32 L33 L35 L44 | L33 L35 L44 L46 | L33 L34 L35 L46 | L36 L37 L39 L48 | L37 L39 L48 L50 | L37 L38 L39 L50 makes body 2 at (-61.1667, 29.8, 49.5667) makes body 3 at (-66.3, 0.8, 49.5667) makes body 4 at (-61.1667, -28.2, 49.5667)
extrude "Extrude5" add sketch "Sketch3" along normal blind 12 from surface at 0.5 contours L31 L40 L42 L43 | L29 L40 L41 L42 | L35 L44 L46 L47 | L33 L44 L45 L46 | L39 L48 L50 L51 | L37 L48 L49 L50 bodies 3 2 4
extrude "Extrude6" add sketch "Sketch3" along normal blind 5.4 separate body contours L16 L17 L18 L19 | L24 L25 L26 L27 makes body 5 at (28.3333, -23.1333, 43) makes body 6 at (67, 10.5333, 43)
extrude "Extrude7" add sketch "Sketch3" along normal blind 5.4 separate body contours L52 L53 L54 L55 A2 A3 A4 A5 | L56 L57 L58 L59 L60 L61 | L62 L63 L64 L65 L66 L67 | L92 A6 L93 A7 L94 A8 L95 A9 makes body 7 at (57.2691, -29.7959, 43) makes body 8 at (70.8635, -29.2416, 43) makes body 9 at (81.3452, -29.7495, 43)
extrude "Extrude8" add sketch "Sketch3" along normal blind 12 separate body contours L8 L96 L97 L99 | L8 L10 L97 L98 L99 makes body 10
extrude "Extrude9" add sketch "Sketch3" along normal blind 11 separate body contours A0 makes body 11
extrude "Extrude10" add sketch "Sketch3" along normal blind 5 separate body contours A1 makes body 12
extrude "Extrude11" add sketch "Sketch3" along normal blind 4.5 separate body contours L12 L13 L14 L15 makes body 13
extrude "Extrude12" cut sketch "Sketch3" against normal blind 1 contours L20 L21 L22 L23 bodies 1 4 2 3 13 12 11 10 9 8 7 6 5
sketch "Sketch4" plane through (0, 0, 43) normal (0, 0, 1) x (-1, 0, 0)
  line L0 (-97.7934, 11.596) -> (-97.7934, 14.801)
  line L1 (-97.7934, 14.801) -> (-90.2257, 14.801)
  line L2 (-90.2257, 14.801) -> (-90.2257, 11.596)
  line L3 (-90.2257, 11.596) -> (-97.7934, 11.596)
  line L4 (107.2, -48.2) -> (107.2, 48.2)
  line L5 (107.2, 48.2) -> (-107.2, 48.2)
  line L6 (-107.2, 48.2) -> (-107.2, -48.2)
  line L7 (-107.2, -48.2) -> (107.2, -48.2)
  line L8 (88.6, -90.5) -> (-73.9, -90.5)
  dimension "d71" = 162.5
  constraint horizontal L8
  measures "d71" distance of L8.start L8.end
equation "d10 = 6.7 mm - d9 / 2"
equation "d16 = 6.42 mm - d14 / 2"
equation "d28 = d26"
equation "d29 = d25"
equation "d34 = d26"
equation "d45 = d41"
equation "d46 = d42"

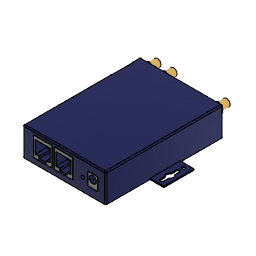
design "Quartzlite Router"
Autodesk Fusion 360 part; units mm, degrees
sketch "Sketch1" plane through (0, 0, 0) normal (0, 0, 1) x (1, 0, 0)
  line L0 (36, 51) -> (-36, 51)
  line L1 (-36, 51) -> (-36, -51)
  line L2 (-36, -51) -> (36, -51)
  line L3 (36, -51) -> (36, 51)
  line L4 (36, 51) -> (-36, -51) construction
  line L5 (-36, 51) -> (36, -51) construction
  line L6 (-48.1, 13.7) -> (-36, 13.7)
  line L7 (-36, 13.7) -> (-36, -12.6)
  line L8 (-36, -12.6) -> (-48.1, -12.6)
  line L9 (-48.1, -12.6) -> (-48.1, 13.7)
  line L10 (0, 0) -> (-36, 0) construction
  line L11 (-44.1, 5.15) -> (-44.1, -8.65)
  arc A0 (-44.1, -8.65) -> (-41.1, -8.65) centre (-42.6, -8.65) ccw
  line L12 (-41.1, -8.65) -> (-41.1, 5.15)
  arc A1 (-41.1, 5.15) -> (-44.1, 5.15) centre (-42.6, 5.15) ccw
  line L13 (-42.6, 5.15) -> (-42.6, -8.65) construction
  circle A2 centre (-42.6, -1.75) radius 2.94
  circle A3 centre (-42.6, 10) radius 1.5
  line L14 (0, 0) -> (0, 51) construction
  arc A4 (44.1, 5.15) -> (41.1, 5.15) centre (42.6, 5.15) ccw
  line L15 (36, 13.7) -> (36, -12.6)
  line L16 (48.1, 13.7) -> (36, 13.7)
  line L17 (44.1, 5.15) -> (44.1, -8.65)
  line L18 (42.6, 5.15) -> (42.6, -8.65) construction
  line L19 (36, -12.6) -> (48.1, -12.6)
  arc A5 (41.1, -8.65) -> (44.1, -8.65) centre (42.6, -8.65) ccw
  circle A6 centre (42.6, -1.75) radius 2.94
  circle A7 centre (42.6, 10) radius 1.5
  line L20 (48.1, -12.6) -> (48.1, 13.7)
  line L21 (41.1, -8.65) -> (41.1, 5.15)
  point P0 (36, 0)
  dimension "d1" = 102
  dimension "d2" = 72
  dimension "d3" = 48.1
  dimension "d4" = 26.3
  dimension "d5" = 3
  dimension "d6" = 13.8
  dimension "d7" = 3.95
  dimension "d8" = 5.88
  dimension "d9" = 5.5
  dimension "d10" = 3
  dimension "d11" = 3.7
  dimension "d12" = 38.4
  constraint horizontal L0
  constraint perpendicular L0 L1
  constraint parallel L0 L2
  constraint parallel L1 L3
  constraint coincident L4 L10.start
  constraint coincident L5 L10.start
  constraint coincident L10.start L14.start
  constraint horizontal L6
  constraint vertical L7
  constraint horizontal L8
  constraint vertical L9
  constraint coincident L1 L7.end
  constraint midpoint L1 L10.end
  constraint tangent L11 A0
  constraint tangent A0 L12
  constraint parallel L11 L12
  constraint tangent L12 A1
  constraint tangent L11 A1
  constraint parallel L1 L13
  constraint midpoint L13 A2.centre
  constraint coincident L13 A3.centre
  constraint midpoint L0 L14.end
  constraint symmetric L6.start L14 L16.start
  constraint symmetric L6.end L14 L15.start
  constraint symmetric L7.end L14 L15.end
  constraint symmetric L8.end L14 L19.end
  constraint symmetric L10.end L14 P0
  constraint symmetric L11.start L14 A4.start
  constraint symmetric L11.end L14 L17.end
  constraint symmetric A0.end L14 A5.start
  constraint symmetric L12.end L14 A4.end
  constraint symmetric A0 L14 A5
  constraint symmetric A1 L14 A4
  constraint symmetric A2 L14 A6
  constraint symmetric A3 L14 A7
  measures "d1" distance of L0.end L1.end
  measures "d2" distance of L0.start L0.end
  measures "d3" distance of L10.start L9
  measures "d4" distance of L6 L8
  measures "d5" distance of L11 L12
  measures "d6" distance of A1.centre A0.centre
  measures "d7" distance of L8 A0.centre
  measures "d8" diameter of A2
  measures "d9" distance of L9 L13
  measures "d10" diameter of A3
  measures "d11" distance of L6 A3.centre
  measures "d12" distance of L2 L8
extrude "Extrude1" add sketch "Sketch1" along normal blind 24.7 contours L0 L1 L2 L3 L7 L15 makes body 1
extrude "Extrude2" add sketch "Sketch1" along normal blind 1 contours L3 L15 L16 L19 L20 | L1 L6 L7 L8 L9 bodies 1
sketch "Sketch2" plane through (0, 51, 0) normal (0, 1, 0) x (-1, 0, 0)
  line L0 (-36, 0) -> (36, 0)
  line L1 (36, 0) -> (36, 24.7)
  line L2 (36, 24.7) -> (-36, 24.7)
  line L3 (-36, 24.7) -> (-36, 0)
  line L4 (30.1, 23.3188) -> (26.1, 21.0094)
  line L5 (26.1, 21.0094) -> (26.1, 16.3906)
  line L6 (26.1, 16.3906) -> (30.1, 14.0812)
  line L7 (30.1, 14.0812) -> (34.1, 16.3906)
  line L8 (34.1, 16.3906) -> (34.1, 21.0094)
  line L9 (34.1, 21.0094) -> (30.1, 23.3188)
  circle A0 centre (30.1, 18.7) radius 3.1
  circle A1 centre (-17.1, 12.5) radius 1.5
  circle A2 centre (-11.1, 12.5) radius 1.5
  circle A3 centre (-5.1, 12.5) radius 1.5
  circle A4 centre (6.9, 12.5) radius 1.5
  circle A5 centre (6.9, 12.5) radius 1.5
  line L10 (-17.1, 12.5) -> (6.9, 12.5) construction
  circle A6 centre (0.9, 12.5) radius 1.5
  line L11 (-36, 0) -> (36, 0)
  circle A7 centre (16.1, 18.7) radius 3.1
  line L12 (30.1, 18.7) -> (-30, 18.7) construction
  circle A8 centre (-30, 18.7) radius 3.1
  line L13 (16.1, 23.3188) -> (12.1, 21.0094)
  line L14 (12.1, 21.0094) -> (12.1, 16.3906)
  line L15 (12.1, 16.3906) -> (16.1, 14.0812)
  line L16 (16.1, 14.0812) -> (20.1, 16.3906)
  line L17 (20.1, 16.3906) -> (20.1, 21.0094)
  line L18 (20.1, 21.0094) -> (16.1, 23.3188)
  line L19 (-30, 23.3188) -> (-34, 21.0094)
  line L20 (-34, 21.0094) -> (-34, 16.3906)
  line L21 (-34, 16.3906) -> (-30, 14.0812)
  line L22 (-30, 14.0812) -> (-26, 16.3906)
  line L23 (-26, 16.3906) -> (-26, 21.0094)
  line L24 (-26, 21.0094) -> (-30, 23.3188)
  point P0 (30.1, 18.7)
  point P1 (16.1, 18.7)
  point P2 (-30, 18.7)
  dimension "d17" = 4
  dimension "d18" = 6.2
  dimension "d20" = 3
  dimension "d21" = 3
  dimension "d22" = 3
  dimension "d23" = 3
  dimension "d24" = 3
  dimension "d25" = 3
  dimension "d26" = 6
  dimension "d27" = 6
  dimension "d28" = 6
  dimension "d29" = 6
  dimension "d30" = 12.5
  dimension "d31" = 18.9
  dimension "d32" = 5.9
  dimension "d33" = 6
  dimension "d34" = 6.2
  dimension "d35" = 6.2
  dimension "d36" = 4
  dimension "d37" = 4
  dimension "d38" = 6
  dimension "d39" = 14
  constraint coincident P0 A0.centre
  constraint coincident A1.centre L10.start
  constraint coincident A4.centre A5.centre
  constraint horizontal L10
  constraint coincident A4.centre L10
  constraint coincident L10 A6.centre
  constraint coincident A2.centre L10
  constraint coincident A3.centre L10
  constraint parallel L1 L8
  constraint horizontal L12
  constraint coincident P1 L12
  constraint coincident P2 L12.end
  constraint coincident P1 A7.centre
  constraint vertical L23
  constraint vertical L17
  measures "d17" distance of P0 L9
  measures "d18" diameter of A0
  measures "d20" diameter of A1
  measures "d21" diameter of A2
  measures "d22" diameter of A3
  measures "d23" diameter of A4
  measures "d24" diameter of A5
  measures "d25" diameter of A6
  measures "d26" distance of A1.centre A2.centre
  measures "d27" distance of A2.centre A3.centre
  measures "d28" distance of A3.centre A6.centre
  measures "d29" distance of A4.centre A6.centre
  measures "d30" distance of A2.centre L11
  measures "d31" distance of L3 A1.centre
  measures "d32" distance of L1 P0
  measures "d33" distance of L2 P0
  measures "d34" diameter of A7
  measures "d35" diameter of A8
  measures "d36" distance of P1 L18
  measures "d37" distance of P2 L24
  measures "d38" distance of L3 P2
  measures "d39" distance of P0 P1
extrude "Extrude3" add sketch "Sketch2" along normal blind 1.6 separate body contours L4 L5 L6 L7 L8 L9 | A1 | A2 | A3 | A4 A5 | A6 | L13 L14 L15 L16 L17 L18 | L19 L20 L21 L22 L23 L24 makes body 2 at (3.6075, 52.0667, 12.3506) makes body 3 at (-19.1846, 52.0667, 18.3913) makes body 4 at (-33.1846, 52.0667, 18.3913) makes body 5 at (9.6075, 52.0667, 12.3506) makes body 6 at (-2.3925, 52.0667, 12.3506) makes body 7 at (26.9154, 52.0667, 18.3913) makes body 8 at (-8.3925, 52.0667, 12.3506) makes body 9 at (15.6075, 52.0667, 12.3506)
extrude "Extrude4" add sketch "Sketch2" along normal blind 9 separate body contours A0 | A7 | A8 makes body 10 at (26.9039, 57, 18.5455) makes body 11 at (-19.1961, 57, 18.5455) makes body 12 at (-33.1961, 57, 18.5455)